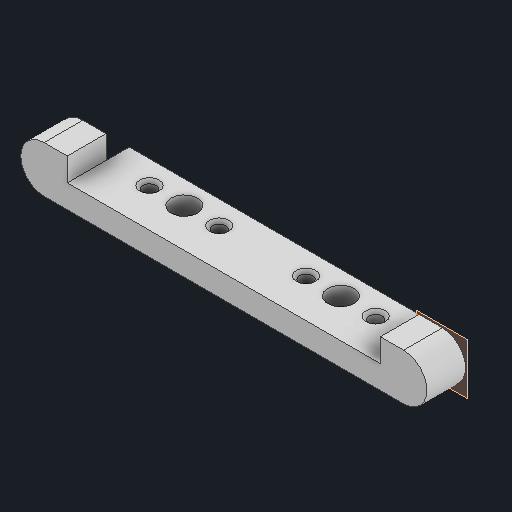
# Autodesk Inventor part: leftfrontmotorwall
Saved by Autodesk Inventor 2026.2 (Build 302298010, 298A)
## iProperties
Created: 2026-09-21
Part Number: leftfrontmotorwall
Material: Generic
Document SubType Name: Modeling
Designer: karol
Density: 1 g/cm^3
Appearance: Default
Author: karol
Autodesk Inventor part; units mm, degrees
ref_plane "YZ Plane" through (0, 0, 0) normal (1, 0, 0) x (0, 1, 0)
ref_plane "XZ Plane" through (0, 0, 0) normal (0, 1, 0) x (-1, 0, 0)
ref_plane "XY Plane" through (0, 0, 0) normal (0, 0, 1) x (1, 0, 0)
sketch "Sketch1" plane through (0, 0, 0) normal (0, 0, 1) x (1, 0, 0)
  line L0 (-58, -60) -> (-60, -60) projected
  line L1 (-60, -60) -> (-60, -39.5) projected
  line L2 (-60, -39.5) -> (-58, -39.5) projected
  line L3 (-58, -39.5) -> (-58, -60) projected
  line L4 (49.6, 30) -> (51.6, 30) projected
  line L5 (51.6, 30) -> (51.6, 9.5) projected
  line L6 (51.6, 9.5) -> (49.6, 9.5) projected
  line L7 (49.6, 9.5) -> (49.6, 30) projected
  line L8 (-58, 39.5) -> (-60, 39.5) projected
  line L9 (-60, 39.5) -> (-60, 60) projected
  line L10 (-60, 60) -> (-58, 60) projected
  line L11 (-58, 60) -> (-58, 39.5) projected
  line L12 (-21.6, -39.5) -> (-19.6, -39.5) projected
  line L13 (-19.6, -39.5) -> (-19.6, -60) projected
  line L14 (-19.6, -60) -> (-21.6, -60) projected
  line L15 (-21.6, -60) -> (-21.6, -39.5) projected
  line L16 (51.6, -30) -> (49.6, -30) projected
  line L17 (49.6, -30) -> (49.6, -9.5) projected
  line L18 (49.6, -9.5) -> (51.6, -9.5) projected
  line L19 (51.6, -9.5) -> (51.6, -30) projected
  line L20 (-21.6, 60) -> (-19.6, 60) projected
  line L21 (-19.6, 60) -> (-19.6, 39.5) projected
  line L22 (-19.6, 39.5) -> (-21.6, 39.5) projected
  line L23 (-21.6, 39.5) -> (-21.6, 60) projected
  line L24 (90, -35) -> (90, 35) projected
  line L25 (90, 35) -> (49.6, 35) projected
  line L26 (49.6, 35) -> (49.6, 60) projected
  line L27 (49.6, 60) -> (90, 60) projected
  line L28 (90, 60) -> (90, 90) projected
  line L29 (90, 90) -> (-19.6, 90) projected
  line L30 (-19.6, 90) -> (-19.6, 65) projected
  line L31 (-19.6, 65) -> (-60, 65) projected
  line L32 (-60, 65) -> (-60, 90) projected
  line L33 (-60, 90) -> (-90, 90) projected
  line L34 (-90, 90) -> (-90, -90) projected
  line L35 (-90, -90) -> (-60, -90) projected
  line L36 (-60, -90) -> (-60, -65) projected
  line L37 (-60, -65) -> (-19.6, -65) projected
  line L38 (-19.6, -65) -> (-19.6, -90) projected
  line L39 (-19.6, -90) -> (90, -90) projected
  line L40 (90, -90) -> (90, -60) projected
  line L41 (90, -60) -> (49.6, -60) projected
  line L42 (49.6, -60) -> (49.6, -35) projected
  line L43 (49.6, -35) -> (90, -35) projected
  line L44 (86, -32) -> (73.8, -32) projected
  line L45 (73.8, -32) -> (73.8, -7.5) projected
  line L46 (73.8, -7.5) -> (86, -7.5) projected
  line L47 (86, -7.5) -> (86, -32) projected
  line L48 (65.8, -32) -> (53.6, -32) projected
  line L49 (53.6, -32) -> (53.6, -7.5) projected
  line L50 (53.6, -7.5) -> (65.8, -7.5) projected
  line L51 (65.8, -7.5) -> (65.8, -32) projected
  line L52 (86, -86) -> (70.6, -86) projected
  line L53 (70.6, -86) -> (70.6, -69.8) projected
  line L54 (70.6, -69.8) -> (86, -69.8) projected
  line L55 (86, -69.8) -> (86, -86) projected
  line L56 (86, 86) -> (86, 69.8) projected
  line L57 (86, 69.8) -> (70.6, 69.8) projected
  line L58 (70.6, 69.8) -> (70.6, 86) projected
  line L59 (70.6, 86) -> (86, 86) projected
  line L60 (73.8, 32) -> (86, 32) projected
  line L61 (86, 32) -> (86, 7.5) projected
  line L62 (86, 7.5) -> (73.8, 7.5) projected
  line L63 (73.8, 7.5) -> (73.8, 32) projected
  line L64 (65.8, 32) -> (65.8, 7.5) projected
  line L65 (65.8, 7.5) -> (53.6, 7.5) projected
  line L66 (53.6, 7.5) -> (53.6, 32) projected
  line L67 (53.6, 32) -> (65.8, 32) projected
  line L68 (-69.6, -87) -> (-85, -87) projected
  line L69 (-85, -87) -> (-85, -70.8) projected
  line L70 (-85, -70.8) -> (-69.6, -70.8) projected
  line L71 (-69.6, -70.8) -> (-69.6, -87) projected
  line L72 (-56, -62) -> (-56, -37.5) projected
  line L73 (-56, -37.5) -> (-43.8, -37.5) projected
  line L74 (-43.8, -37.5) -> (-43.8, -62) projected
  line L75 (-43.8, -62) -> (-56, -62) projected
  line L76 (-56, 62) -> (-43.8, 62) projected
  line L77 (-43.8, 62) -> (-43.8, 37.5) projected
  line L78 (-43.8, 37.5) -> (-56, 37.5) projected
  line L79 (-56, 37.5) -> (-56, 62) projected
  line L80 (-23.6, 62) -> (-23.6, 37.5) projected
  line L81 (-23.6, 37.5) -> (-35.8, 37.5) projected
  line L82 (-35.8, 37.5) -> (-35.8, 62) projected
  line L83 (-35.8, 62) -> (-23.6, 62) projected
  line L84 (-23.6, -62) -> (-35.8, -62) projected
  line L85 (-35.8, -62) -> (-35.8, -37.5) projected
  line L86 (-35.8, -37.5) -> (-23.6, -37.5) projected
  line L87 (-23.6, -37.5) -> (-23.6, -62) projected
  line L88 (-85, 87) -> (-69.6, 87) projected
  line L89 (-69.6, 87) -> (-69.6, 70.8) projected
  line L90 (-69.6, 70.8) -> (-85, 70.8) projected
  line L91 (-85, 70.8) -> (-85, 87) projected
  line L92 (-19.6, 65) -> (-63, 65)
  line L93 (-63, 65) -> (-63, 62)
  line L94 (-63, 62) -> (-19.6, 62)
  line L95 (-19.6, 62) -> (-19.6, 65)
  line L96 (-63, 62) -> (-60, 62)
  line L97 (-60, 62) -> (-60, 65)
  line L98 (-60, 65) -> (-63, 65)
  line L99 (-63, 65) -> (-63, 62)
  line L100 (-60, 62) -> (-66, 62)
  line L101 (-66, 62) -> (-66, 68)
  line L102 (-66, 68) -> (-60, 68)
  line L103 (-60, 68) -> (-60, 62)
  circle A0 centre (-63, -65) radius 1.5 projected
  circle A1 centre (-16.6, -87) radius 1.5 projected
  circle A2 centre (49.6, -87) radius 1.5 projected
  circle A3 centre (46.6, -60) radius 1.5 projected
  circle A4 centre (87, -63) radius 1.5 projected
  circle A5 centre (46.6, -32) radius 1.5 projected
  circle A6 centre (46.6, 32) radius 1.5 projected
  circle A7 centre (87, 63) radius 1.5 projected
  circle A8 centre (46.6, 60) radius 1.5 projected
  circle A9 centre (49.6, 87) radius 1.5 projected
  circle A10 centre (-16.6, 87) radius 1.5 projected
  circle A11 centre (-16.6, 65) radius 1.5 projected
  circle A12 centre (-63, 65) radius 1.5 projected
  point P0 (0, 0)
  dimension "d0" = 43.4
  dimension "d1" = 6
  dimension "d2" = 6
  constraints: 24 end point, 6 parallel, 3 horizontal, 3 perpendicular
  measures "d0" distance of L94.end L93.end
  measures "d1" distance of L101.end L102.end
  measures "d2" distance of L100.end L101.end
extrude "Extrusion1" add sketch "Sketch1" along normal blind 8 contours L95 L94 L83 L76 L97 L31 | L92 A12 L93 L100 L101 L102 L32 | L97 L94 L93 A12 L92 | A12 L93 L92 | L92 L93 A12
ref_plane "Work Plane1" through (-16.6, 65, 3) normal (0, 0, 1) x (1, 0, 0)
sketch "Sketch2" plane through (-16.6, 65, 3) normal (0, 0, 1) x (1, 0, 0)
  circle A0 centre (0, 0) radius 1.65 projected
  line L0 (0, -3) -> (-3, -3) projected
  line L1 (-3, 3) -> (0, 3) projected
  line L2 (-3, -3) -> (-3, 3) projected
  line L3 (3, 3) -> (-3, 3)
  line L4 (-3, 3) -> (-3, -3)
  line L5 (-3, -3) -> (3, -3)
  line L6 (3, -3) -> (3, 3)
  arc A1 (0, -3) -> (0, 3) centre (0, 0) ccw projected
  point P0 (16.6, -65)
  constraints: 8 end point, 2 parallel, 1 horizontal, 1 perpendicular
extrude "Extrusion2" add sketch "Sketch2" along normal blind 5 contours L0 L2 L1 A1
sketch "Sketch4" plane through (0, 0, 0) normal (0, 0, -1) x (-1, 0, 0)
  line L0 (60, 68) -> (66, 68) projected
  line L1 (66, 62) -> (16.6, 62) projected
  line L2 (60, 68) -> (66, 68)
  line L3 (66, 68) -> (66, 62)
  line L4 (66, 62) -> (60, 62)
  line L5 (60, 62) -> (60, 68)
  line L6 (66, 68) -> (60, 62)
  line L7 (60, 65) -> (60, 68) projected
  line L8 (60, 68) -> (66, 62)
  circle A0 centre (63, 65) radius 2
  point P0 (0, 0)
  point P1 (13.6, 62)
  dimension "d9" = 4
  constraints: 12 end point, 2 parallel, 2 perpendicular, 1 centre point, 1 horizontal, 1 midpoint
  measures "d9" diameter of A0
extrude "Extrusion4" cut sketch "Sketch4" against normal blind 7 contours A0 L6 L8 | L8 L6 A0 | A0 L8 L6 | L8 A0 L6
extrude "Extrusion5" cut sketch "Sketch4" against normal blind 3 contours L8 A0 L6 L5 | L0 L6 A0 L8 | L3 L8 A0 L6 | L1 L6 A0 L8
sketch "Sketch5" plane through (-16.6, 65, 3) normal (0, 0, -1) x (-1, 0, 0)
  circle A0 centre (0, 0) radius 1.65 projected
  circle A1 centre (0, 0) radius 2
  point P0 (-16.6, -65)
  dimension "d14" = 4
  constraints: 1 centre point, 1 coincident
  measures "d14" diameter of A1
extrude "Extrusion6" cut sketch "Sketch5" against normal blind 4
sketch "Sketch6" plane through (0, 0, 8) normal (0, 0, 1) x (1, 0, 0)
  circle A0 centre (-16.6, 65) radius 1.65 projected
  circle A1 centre (-16.6, 65) radius 1.65
  point P0 (0, 0)
  constraints: 1 centre point, 1 coincident
extrude "Extrusion7" add sketch "Sketch6" against normal blind 1
sketch "Sketch7" plane through (-60, 65, 8) normal (0, 1, 0) x (1, 0, 0)
  circle A0 centre (34.8, 5) radius 0.85
  circle A1 centre (25.8, 5) radius 0.85
  circle A2 centre (14.6, 5) radius 0.85
  circle A3 centre (5.6, 5) radius 0.85
  circle A4 centre (10.1, 5) radius 1.7
  circle A5 centre (30.3, 5) radius 1.7
  line L0 (40.4, 8) -> (40.4, 5) projected
  line L1 (0, 8) -> (0, 5) projected
  line L2 (40.4, 8) -> (0, 8) projected
  point P0 (60, 8)
  point P1 (0, 6.5)
  dimension "d19" = 1.7
  dimension "d20" = 1.7
  dimension "d21" = 1.7
  dimension "d22" = 1.7
  dimension "d23" = 3.4
  dimension "d24" = 3.4
  dimension "d25" = 10.1
  dimension "d26" = 4.5
  dimension "d27" = 4.5
  dimension "d28" = 4.5
  dimension "d29" = 4.5
  dimension "d30" = 10.1
  dimension "d31" = 3
  dimension "d32" = 3
  dimension "d33" = 3
  dimension "d34" = 3
  dimension "d35" = 3
  dimension "d36" = 3
  constraints: 6 centre point, 1 midpoint
  measures "d19" diameter of A0
  measures "d20" diameter of A1
  measures "d21" diameter of A2
  measures "d22" diameter of A3
  measures "d23" diameter of A4
  measures "d24" diameter of A5
  measures "d25" distance from line of L0 A5.centre
  measures "d26" distance of A0.centre A5.centre
  measures "d27" distance of A5.centre A1.centre
  measures "d28" distance of A4.centre A2.centre
  measures "d29" distance of A4.centre A3.centre
  measures "d30" horizontal distance of point (0, 6.5) A4.centre
  measures "d31" distance from line of L2 A4.centre
  measures "d32" distance from line of L2 A3.centre
  measures "d33" distance from line of L2 A2.centre
  measures "d34" distance from line of L2 A5.centre
  measures "d35" distance from line of L2 A1.centre
  measures "d36" distance from line of L2 A0.centre
extrude "Extrusion8" cut sketch "Sketch7" against normal blind 10
chamfer "Chamfer1" distance 0.4 angle 45 4 edges at (-26.05, 65, 3) (-35.05, 65, 3) (-46.25, 65, 3) (-55.25, 65, 3)
fillet "Fillet1" radius 0.5 2 edges at (-51.6, 62, 3) (-31.4, 62, 3) inverted yes
fillet "Fillet2" radius 3 2 edges at (-66, 68, 5.5) (-66, 62, 5.5)
body "Solid1"
